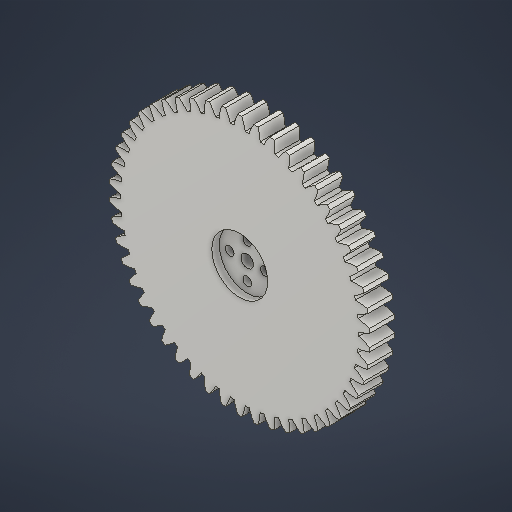
# Autodesk Inventor part: SAFRS-P-0051
Saved by Autodesk Inventor 2026.2 (Build 302298000, 298)
## iProperties
CustomPartVersion: 1
Created: 2025-11-12
Part Number: SAFRS-P-0051
Material: Steel
Document SubType Name: Modeling
Designer: jaewook
Categories: <?xml version="1.0" encoding="UTF-16"?> <MemberInstance><Categories><FamilyTemplate><FamilyTemplateParameter ValueType="xs:double" Id="1" ObjectReferenceKey="da_z" ObjectType="kUserParameterObject"/><FamilyTemplateParameter ValueType="xs:double" Id="2" ObjectReferenceKey="da_b" ObjectType="kUserParameterObject"/><FamilyTemplateParameter ValueType="xs:double" Id="3" ObjectReferenceKey="da_beta" ObjectType="kUserParameterObject"/><FamilyTemplateParameter ValueType="xs:double" Id="4" ObjectReferenceKey="da_da" ObjectType="kUserParameterObject"/><FamilyTemplateParameter ValueType="xs:double" Id="5" ObjectReferenceKey="da_aw" ObjectType="kUserParameterObject"/><FamilyTemplateParameter ValueType="xs:string" Id="6" ObjectReferenceKey="EAIAABAAAACIAQAAAAAAAIAAAAAAAAAA" ObjectType="83910656" SubObjectId="SurfaceGeometry"/></FamilyTemplate><ParamToTemplateMap><ParamToTemplate CategoryParameter="//CategoryParameter[@InternalName='046C89C9-8512-4d59-83FE-43B91F4F132A']" TemplateParameter="1"/><ParamToTemplate CategoryParameter="//CategoryParameter[@InternalName='2552DF32-E462-4b46-AEBF-C6C7768E72AC']" TemplateParameter="2"/><ParamToTemplate CategoryParameter="//CategoryParameter[@InternalName='C9EE641D-15FC-4fae-A226-E94C4372FDD7']" TemplateParameter="3"/><ParamToTemplate><ParamToTemplate CategoryParameter="//CategoryParameter[@InternalName='00B6519A-459B-49c7-AD84-2E56D39A5744']" ConstantValue="0.000000"/></ParamToTemplate><ParamToTemplate><ParamToTemplate CategoryParameter="//CategoryParameter[@InternalName='04B31F0E-C7A6-4894-AA32-9629BEFACF47']" ConstantValue="0.980000"/></ParamToTemplate><ParamToTemplate><ParamToTemplate CategoryParameter="//CategoryParameter[@InternalName='43CBEC2E-7847-49e7-A936-2F7889FCB2D9']" ConstantValue="0.250000"/></ParamToTemplate><ParamToTemplate><ParamToTemplate CategoryParameter="//CategoryParameter[@InternalName='B1EFC894-105D-4ebd-86BF-FA20ED196853']" ConstantValue="0.379900"/></ParamToTemplate><ParamToTemplate><ParamToTemplate CategoryParameter="//CategoryParameter[@InternalName='51175063-3D10-4879-93E8-6246FE8B403D']" ConstantValue="2060000000.000000"/></ParamToTemplate><ParamToTemplate><ParamToTemplate CategoryParameter="//CategoryParameter[@InternalName='A3A52E27-4454-46a9-B0BD-C932399B70AF']" ConstantValue="0.300000"/></ParamToTemplate><ParamToTemplate><ParamToTemplate CategoryParameter="//CategoryParameter[@InternalName='91B76062-C214-41d9-B1B9-14D2AB99603D']" ConstantValue="0.200000"/></ParamToTemplate><ParamToTemplate><ParamToTemplate CategoryParameter="//CategoryParameter[@InternalName='374E806E-8B8A-4dda-A9AA-1039D6500AD2']" ConstantValue="5.000000"/></ParamToTemplate><ParamToTemplate><ParamToTemplate CategoryParameter="//CategoryParameter[@InternalName='2D373A89-B862-43d6-8D0B-0CBF12AB9F6C']" ConstantValue="0.349066"/></ParamToTemplate><ParamToTemplate CategoryParameter="//CategoryParameter[@InternalName='37777632-D6A2-4fac-9D53-DB8ACD95C989']" TemplateParameter="4"/><ParamToTemplate CategoryParameter="//CategoryParameter[@InternalName='FD1017F1-B727-4f7e-9707-0F86F1FF9423']" TemplateParameter="5"/><ParamToTemplate><ParamToTemplate CategoryParameter="//CategoryParameter[@InternalName='9E1B4470-B2D3-4ff1-B813-535BB4CDF51A']" ConstantValue="3520000.000000"/></ParamToTemplate><ParamToTemplate><ParamToTemplate CategoryParameter="//CategoryParameter[@InternalName='F8452263-BFF6-458c-9FB1-07C4B99E95CD']" ConstantValue="11400000.000000"/></ParamToTemplate><ParamToTemplate><ParamToTemplate CategoryParameter="//CategoryParameter[@InternalName='3E3BB259-FD49-497f-8171-6EBC954A3479']" ConstantValue="2.000000"/></ParamToTemplate><ParamToTemplate CategoryParameter="//CategoryParameter[@InternalName='27C3BAF2-7550-4e4b-AE2C-0DB134B7D9B7']" TemplateParameter="6"/></ParamToTemplateMap><Category DisplayName="Gear" InternalName="DC85795E-93AB-48d5-8EEE-5A27447B64BD" Mnemonic="Gear"><CategoryParameter DisplayName="z" InternalName="046C89C9-8512-4d59-83FE-43B91F4F132A" Mnemonic="z"/><CategoryParameter DisplayName="b" InternalName="2552DF32-E462-4b46-AEBF-C6C7768E72AC" Mnemonic="b"/><CategoryParameter DisplayName="||b|" InternalName="C9EE641D-15FC-4fae-A226-E94C4372FDD7" Mnemonic="beta"/><CategoryParameter DisplayName="x" InternalName="00B6519A-459B-49c7-AD84-2E56D39A5744" Mnemonic="x"/><CategoryParameter DisplayName="a*" InternalName="04B31F0E-C7A6-4894-AA32-9629BEFACF47" Mnemonic="a"/><CategoryParameter DisplayName="c*" InternalName="43CBEC2E-7847-49e7-A936-2F7889FCB2D9" Mnemonic="c"/><CategoryParameter DisplayName="r|.f|*" InternalName="B1EFC894-105D-4ebd-86BF-FA20ED196853" Mnemonic="rf"/><CategoryParameter DisplayName="E" InternalName="51175063-3D10-4879-93E8-6246FE8B403D" Mnemonic="E"/><CategoryParameter DisplayName="||m|" InternalName="A3A52E27-4454-46a9-B0BD-C932399B70AF" Mnemonic="mi"/><Category DisplayName="SpurGear" InternalName="26C5A22E-A91E-4dfd-A3B3-23CCAFAE1764" Mnemonic="SpurGear"><CategoryParameter DisplayName="m" InternalName="91B76062-C214-41d9-B1B9-14D2AB99603D" Mnemonic="m"/><CategoryParameter DisplayName="P" InternalName="374E806E-8B8A-4dda-A9AA-1039D6500AD2" Mnemonic="PP"/><CategoryParameter DisplayName="||a|" InternalName="2D373A89-B862-43d6-8D0B-0CBF12AB9F6C" Mnemonic="alpha"/><CategoryParameter DisplayName="d|.a|" InternalName="37777632-D6A2-4fac-9D53-DB8ACD95C989" Mnemonic="da"/><CategoryParameter DisplayName="a|.w|" InternalName="FD1017F1-B727-4f7e-9707-0F86F1FF9423" Mnemonic="aw"/><CategoryParameter DisplayName="||s||.Flim|" InternalName="9E1B4470-B2D3-4ff1-B813-535BB4CDF51A" Mnemonic="sFlim"/><CategoryParameter DisplayName="||s||.Hlim|" InternalName="F8452263-BFF6-458c-9FB1-07C4B99E95CD" Mnemonic="sHlim"/><CategoryParameter DisplayName="유형" InternalName="3E3BB259-FD49-497f-8171-6EBC954A3479" Mnemonic="type"/><CategoryParameter DisplayName="PitchDiameter" InternalName="27C3BAF2-7550-4e4b-AE2C-0DB134B7D9B7" Mnemonic="IDS_PITCHDIAM"/></Category></Category></Categories></MemberInstance>
Density: 1 g/cm^3
Appearance: Steel
Author: jaewook
Title: Spur Gear 15T
Autodesk Inventor part; units mm, degrees
sketch "Sketch1" plane through (0, 0, 0) normal (0, 0, 1) x (1, 0, 0)
  circle A0 centre (0, 0) radius 51.96
  dimension "d0" = 103.92
  constraints: 1 centre point
  measures "d0" diameter of A0
extrude "Extrusion1" add sketch "Sketch1" along normal blind 10
ref_plane "Work Plane2" through (0, 0, 5) normal (0, 0, 1) x (1, 0, 0)
sketch "Sketch2" plane through (0, 0, 0) normal (0, 0, -1) x (-1, 0, 0)
  circle A0 centre (0, 0) radius 51.96 projected
  circle A1 centre (0, 0) radius 50
  dimension "d3" = 100
  constraints: 1 centre point, 1 coincident
  measures "d3" diameter of A1
surface extrude "피치 지름" sketch "Sketch2" against normal through all shown no curves A1
ref_plane "Work Plane8" through (0, 0, 0) normal (0.9980267, 0.0627905, 0) x (0, 0, 1)
ref_plane "Work Plane9" through (0, 0, 0) normal (1, 0, 0) x (0, 1, 0)
spur gear teeth "스퍼 기어" teeth 50 pitch diameter 100 tip diameter 103.92 root diameter 95.08 face width 10 start plane through (0, 0, 0) normal (0, 0, -1) x (-1, 0, 0)
sketch "스케치3" plane through (0, 0, 10) normal (0, 0, 1) x (1, 0, 0)
  arc A0 (-5.7018, 51.6462) -> (-7.3212, 51.4416) centre (0, 0) ccw projected
  circle A1 centre (0, 0) radius 3.15
  circle A2 centre (0, 0) radius 11.15
  dimension "d49" = 6.3
  dimension "d50" = 22.3
  constraints: 2 centre point, 2 coincident
  measures "d49" diameter of A1
  measures "d50" diameter of A2
extrude "돌출2" cut sketch "스케치3" against normal blind 3 contours A1 | A2
sketch "스케치4" plane through (0, 0, 7) normal (0, 0, 1) x (1, 0, 0)
  circle A0 centre (0, 0) radius 11.15 projected
  circle A1 centre (0, 0) radius 2.5
  circle A2 centre (0, 7) radius 1.75
  circle A3 centre (-7, 0) radius 1.75
  circle A4 centre (0, -7) radius 1.75
  circle A5 centre (7, 0) radius 1.75
  circle A6 centre (0, 0) radius 3
  dimension "d53" = 5
  dimension "d54" = 3.5
  dimension "d58" = 360
  dimension "d60" = 6
  dimension "d65" = 7
  constraints: 6 centre point, 2 coincident, 1 vertical alignment, 9 other
  measures "d53" diameter of A1
  measures "d54" diameter of A2
  measures "d60" diameter of A6
  measures "d65" distance of A0.centre A2.centre
sketch "스케치6" plane through (0, 0, 0) normal (0, 0, -1) x (-1, 0, 0)
  arc A0 (9.6405, 46.5523) -> (8.1735, 46.8321) centre (0, 0) ccw projected
  circle A1 centre (0, 0) radius 14.5
  dimension "d73" = 29
  constraints: 1 centre point, 1 coincident
  measures "d73" diameter of A1
extrude "돌출6" add sketch "스케치6" along normal blind 3 draft -40
extrude "돌출3" cut sketch "스케치4" against normal through all contours A2 | A3 | A4 | A5
sketch "스케치5" plane through (0, 0, -3) normal (0, 0, -1) x (-1, 0, 0)
  arc A0 (7.3212, 51.4416) -> (5.7018, 51.6462) centre (0, 0) ccw projected
  circle A1 centre (0, -7) radius 3.6
  circle A2 centre (7, 0) radius 3.6
  circle A3 centre (0, 7) radius 3.6
  circle A4 centre (-7, 0) radius 3.6
  circle A5 centre (0, -7) radius 1.75 projected
  circle A6 centre (7, 0) radius 1.75 projected
  circle A7 centre (-7, 0) radius 1.75 projected
  circle A8 centre (0, 7) radius 1.75 projected
  circle A9 centre (0, 0) radius 11.9827 projected
  dimension "d66" = 7.2
  dimension "d69" = 360
  constraints: 4 centre point, 1 coincident, 9 other
  measures "d66" diameter of A1
extrude "돌출5" cut sketch "스케치5" against normal blind 3 from surface at 0 contours A1 | A2 | A3 | A4 | A5 | A6 | A7 | A8
extrude "돌출4" cut sketch "스케치4" against normal through all contours A1
equation "\"d0\" = da_da"
equation "\"d1\" = da_b"
equation "\"d3\" = da_d"
equation "\"da_da\" = 103.92"
equation "\"da_b\" = 10"
equation "\"da_d\" = 100"
body "Solid1"
body "Srf1"
